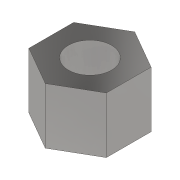
# Autodesk Inventor part: M3_nut
Saved by Autodesk Inventor 2022 (Build 260153000, 153)
## iProperties
Created: 2022-10-12
Part Number: M3_nut
Material: Generic
Document SubType Name: Modeling
Designer: dell
Density: 1 g/cm^3
Appearance: Steel - Polished
Author: dell
Autodesk Inventor part; units mm, degrees
ref_plane "YZ Plane" through (0, 0, 0) normal (1, 0, 0) x (0, 1, 0)
ref_plane "XZ Plane" through (0, 0, 0) normal (0, 1, 0) x (-1, 0, 0)
ref_plane "XY Plane" through (0, 0, 0) normal (0, 0, 1) x (1, 0, 0)
sketch "Sketch1" plane through (0, 0, 0) normal (0, 1, 0) x (-1, 0, 0)
  line L0 (0, -3.1177) -> (-2.7, -1.5588)
  line L1 (-2.7, -1.5588) -> (-2.7, 1.5588)
  line L2 (-2.7, 1.5588) -> (0, 3.1177)
  line L3 (0, 3.1177) -> (2.7, 1.5588)
  line L4 (2.7, 1.5588) -> (2.7, -1.5588)
  line L5 (2.7, -1.5588) -> (0, -3.1177)
  circle A0 centre (0, 0) radius 1.5
  dimension "d0" = 5.4
  dimension "d1" = 3
  constraints: 12 end point, 2 coincident, 1 centre point, 13 other
  measures "d0" distance between parallel lines of L1 L4
  measures "d1" diameter of A0
extrude "Extrusion1" add sketch "Sketch1" along normal blind 3.9
body "Solid1"
